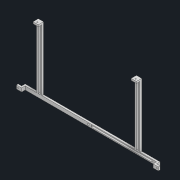
# Autodesk Inventor part: Bancada
Saved by Autodesk Inventor 2021 (Build 250183000, 183)
## iProperties
Created: 2021-04-19
Part Number: Bancada
Material: Genérico
Document SubType Name: Modeling
Designer: carlo
Density: 1 g/cm^3
Appearance: Valor por defecto
Mass: 32.5704 g
Surface Area: 255.981 cm^2
Volume: 32.5704 cm^3
Author: carlo
Autodesk Inventor part; units mm, degrees
ref_plane "YZ Plane" through (0, 0, 0) normal (1, 0, 0) x (0, 1, 0)
ref_plane "XZ Plane" through (0, 0, 0) normal (0, 1, 0) x (-1, 0, 0)
ref_plane "XY Plane" through (0, 0, 0) normal (0, 0, 1) x (1, 0, 0)
sketch "Boceto1" plane through (0, 0, 0) normal (0, 0, 1) x (1, 0, 0)
  line L0 (5, -5) -> (165, -5)
  line L1 (165, -2.5) -> (8, -2.5)
  line L2 (8, -2.5) -> (8, 2.5)
  line L3 (8, 2.5) -> (165, 2.5)
  line L4 (140, 5) -> (142.5, 5)
  line L5 (142.5, 5) -> (137.5, 5)
  line L6 (137.5, 5) -> (137.5, 180)
  line L7 (142.5, 180) -> (142.5, 5)
  line L8 (132.5, 185) -> (147.5, 185)
  line L9 (147.5, 185) -> (147.5, 5)
  line L10 (142.5, 5) -> (137.5, 5)
  line L11 (132.5, 5) -> (132.5, 185)
  line L12 (137.5, 180) -> (142.5, 180)
  line L13 (147.5, 5) -> (165, 5)
  line L14 (0, 5) -> (132.5, 5)
  line L15 (137.5, 5) -> (142.5, 5)
  arc A0 (-165, 5) -> (-165, -5) centre (-165, 0) ccw
  line L16 (5, -5) -> (-165, -5)
  line L17 (-140, 5) -> (-142.5, 5)
  line L18 (-142.5, 5) -> (-137.5, 5)
  line L19 (-137.5, 5) -> (-137.5, 180)
  line L20 (-142.5, 180) -> (-142.5, 5)
  line L21 (-132.5, 185) -> (-147.5, 185)
  line L22 (-147.5, 185) -> (-147.5, 5)
  line L23 (-142.5, 5) -> (-137.5, 5)
  line L24 (-132.5, 5) -> (-132.5, 185)
  line L25 (-137.5, 180) -> (-142.5, 180)
  line L26 (-147.5, 5) -> (-165, 5)
  line L27 (0, 5) -> (-132.5, 5)
  line L28 (-137.5, 5) -> (-142.5, 5)
  line L29 (0, 0) -> (-5, 0) construction
  circle A1 centre (0, 0) radius 2.5
  arc A2 (180, -2.5) -> (180, 2.5) centre (180, 0) ccw
  line L30 (180, 5) -> (165, 5)
  line L31 (165, 2.5) -> (180, 2.5)
  line L32 (165, -2.5) -> (180, -2.5)
  line L33 (165, -5) -> (180, -5)
  arc A3 (180, -5) -> (180, 5) centre (180, 0) ccw
  dimension "d13" = 15
  dimension "d17" = 180
  dimension "d18" = 175
  dimension "d31" = 10
  dimension "d36" = 5
  dimension "d40" = 5
  constraints: 68 end point, 8 parallel, 6 horizontal, 6 point on circle, 4 centre point, 4 perpendicular, 2 coincident, 2 tangent
  measures "d13" distance of L9.end L11.start
  measures "d17" distance of L11.start L8.start
  measures "d18" distance between parallel lines of L14 L12
  measures "d31" distance between parallel lines of L27 L16
  measures "d36" diameter of A1
  measures "d40" diameter of A2
extrude "Extrusión1" add sketch "Boceto1" along normal blind 5
sketch "Sketch4" plane through (0, 0, 5) normal (0, 0, 1) x (1, 0, 0)
  line L0 (-132.5, 185) -> (-147.5, 185) projected
  line L1 (-132.5, 5) -> (-132.5, 185) projected
  line L2 (-147.5, 185) -> (-132.5, 185)
  line L3 (-132.5, 185) -> (-132.5, 180)
  line L4 (-132.5, 180) -> (-147.5, 180)
  line L5 (-147.5, 180) -> (-147.5, 185)
  line L6 (180, 5) -> (147.5, 5) projected
  line L7 (147.5, 5) -> (147.5, 185) projected
  line L8 (147.5, 185) -> (132.5, 185) projected
  line L9 (132.5, 185) -> (132.5, 5) projected
  line L10 (132.5, 5) -> (-132.5, 5) projected
  line L11 (-132.5, 5) -> (-132.5, 185) projected
  line L12 (-132.5, 185) -> (-147.5, 185) projected
  line L13 (-147.5, 185) -> (-147.5, 5) projected
  line L14 (-147.5, 5) -> (-165, 5) projected
  arc A0 (-165, 5) -> (-165, -5) centre (-165, 0) ccw projected
  line L15 (-165, -5) -> (180, -5) projected
  line L16 (-142.5, 5) -> (-142.5, 180) projected
  line L17 (-142.5, 180) -> (-137.5, 180) projected
  line L18 (-137.5, 180) -> (-137.5, 5) projected
  line L19 (-137.5, 5) -> (-142.5, 5) projected
  line L20 (142.5, 180) -> (142.5, 5) projected
  line L21 (142.5, 5) -> (137.5, 5) projected
  line L22 (137.5, 5) -> (137.5, 180) projected
  line L23 (137.5, 180) -> (142.5, 180) projected
  line L24 (132.5, 185) -> (147.5, 185)
  line L25 (147.5, 185) -> (147.5, 180)
  line L26 (147.5, 180) -> (132.5, 180)
  line L27 (132.5, 180) -> (132.5, 185)
  arc A1 (180, -5) -> (180, 5) centre (180, 0) ccw projected
  point P0 (0, 0)
  dimension "d26" = 5
  constraints: 16 end point, 4 parallel, 2 horizontal, 2 perpendicular, 2 point on line
  measures "d26" distance of L2.end L3.end
extrude "Extrusion3" add sketch "Sketch4" along normal blind 10 contours L1 L4 L5 L0 | L9 L8 L7 L26 L23
sketch "Sketch5" plane through (0, 0, 5) normal (0, 0, 1) x (1, 0, 0)
  line L0 (180, -2.5) -> (8, -2.5) projected
  line L1 (8, -2.5) -> (8, 2.5) projected
  line L2 (8, 2.5) -> (180, 2.5) projected
  arc A0 (180, -2.5) -> (180, 2.5) centre (180, 0) ccw projected
  circle A1 centre (0, 0) radius 2.5 projected
  line L3 (147.5, 180) -> (142.5, 180) projected
  line L4 (142.5, 180) -> (142.5, 5) projected
  line L5 (142.5, 5) -> (137.5, 5) projected
  line L6 (137.5, 5) -> (137.5, 180) projected
  line L7 (137.5, 180) -> (132.5, 180) projected
  line L8 (132.5, 180) -> (132.5, 5) projected
  line L9 (132.5, 5) -> (-132.5, 5) projected
  line L10 (-132.5, 5) -> (-132.5, 180) projected
  line L11 (-132.5, 180) -> (-137.5, 180) projected
  line L12 (-137.5, 180) -> (-137.5, 5) projected
  line L13 (-137.5, 5) -> (-142.5, 5) projected
  line L14 (-142.5, 5) -> (-142.5, 180) projected
  line L15 (-142.5, 180) -> (-147.5, 180) projected
  line L16 (-147.5, 180) -> (-147.5, 5) projected
  line L17 (-147.5, 5) -> (-165, 5) projected
  arc A2 (-165, 5) -> (-165, -5) centre (-165, 0) ccw projected
  line L18 (-165, -5) -> (180, -5) projected
  arc A3 (180, -5) -> (180, 5) centre (180, 0) ccw projected
  line L19 (180, 5) -> (147.5, 5) projected
  line L20 (147.5, 5) -> (147.5, 180) projected
  arc A4 (-165, 5) -> (-165, -5) centre (-165, 0) ccw projected
  line L21 (-165, -5) -> (-185, -5)
  line L22 (-185, -5) -> (-185, 5)
  line L23 (-185, 5) -> (-165, 5)
  line L24 (-165, 5) -> (-165, -5)
  arc A5 (180, -5) -> (180, 5) centre (180, 0) ccw projected
  line L25 (180, 5) -> (200, 5)
  line L26 (200, 5) -> (200, -5)
  line L27 (200, -5) -> (180, -5)
  dimension "d42" = 20
  dimension "d45" = 20
  constraints: 14 end point, 3 perpendicular, 2 horizontal, 2 parallel
  measures "d42" distance of L22.end L23.end
  measures "d45" distance of L19.start L25.end
extrude "Extrusion4" add sketch "Sketch5" against normal up to surface (5 mm away) contours L25 L26 L27 A3 | L21 L22 L23 A2 | A2 L24
sketch "Sketch6" plane through (0, 0, 5) normal (0, 0, 1) x (1, 0, 0)
  line L0 (-147.5, 180) -> (-132.5, 180) projected
  line L1 (-132.5, 180) -> (-132.5, 185) projected
  line L2 (-132.5, 185) -> (-147.5, 185) projected
  line L3 (-147.5, 185) -> (-147.5, 180) projected
  line L4 (-147.5, 5) -> (-185, 5) projected
  line L5 (200, -5) -> (-185, -5) projected
  line L6 (-185, 5) -> (-180, 5)
  line L7 (-180, 5) -> (-180, -5)
  line L8 (-180, -5) -> (-185, -5)
  line L9 (-185, -5) -> (-185, 5)
  line L10 (200, -5) -> (200, 5) projected
  line L11 (200, 5) -> (195, 5)
  line L12 (195, 5) -> (195, -5)
  line L13 (195, -5) -> (200, -5)
  line L14 (200, -5) -> (200, 5)
  point P0 (0, 0)
  dimension "d46" = 15
  dimension "d47" = 5
  dimension "d48" = 5
  dimension "d49" = 5
  dimension "d50" = 10
  constraints: 16 end point, 4 parallel, 2 horizontal, 2 perpendicular, 1 point on line
  measures "d46" distance of L1.end L2.end
  measures "d47" distance of L0.end L1.end
  measures "d48" distance of L7.end L8.end
  measures "d49" distance of L13.end L12.end
  measures "d50" distance of L12.end L11.end
extrude "Extrusion5" add sketch "Sketch6" along normal up to surface (10 mm away) contours L7 L5 L9 L4 | L12 L11 L10 L5
sketch "Sketch7" plane through (-185, -5, 0) normal (-1, 0, 0) x (0, 0, 1)
  line L0 (15, 0) -> (15, 10) projected
  line L1 (0, 0) -> (15, 0) projected
  line L2 (15, 10) -> (10, 10)
  line L3 (10, 10) -> (10, 0)
  line L4 (10, 0) -> (15, 0)
  line L5 (15, 0) -> (15, 10)
  point P0 (0, 5)
  dimension "d53" = 5
  constraints: 8 end point, 2 parallel, 1 horizontal, 1 perpendicular, 1 point on line
  measures "d53" distance of L4.end L3.end
extrude "Extrusion6" add sketch "Sketch7" along normal blind 10
sketch "Sketch8" plane through (200, -5, 0) normal (1, 0, 0) x (0, 0, -1)
  line L0 (-10, 10) -> (-10, 0) projected
  line L1 (-10, 0) -> (-15, 0) projected
  line L2 (-15, 0) -> (-15, 10) projected
  line L3 (-15, 10) -> (-10, 10) projected
  point P0 (0, 5)
extrude "Extrusion7" add sketch "Sketch8" along normal blind 10
sketch "Sketch9" plane through (-180, -5, 15) normal (0, 0, 1) x (1, 0, 0)
  line L0 (32.5, 10) -> (-5, 10) projected
  line L1 (0, 0) -> (375, 0) projected
  line L2 (-5, 0) -> (-5, 10) projected
  line L3 (0, 0) -> (-15, 0) projected
  line L4 (0, 10) -> (0, 0) projected
  line L5 (0, 10) -> (-15, 10) projected
  line L6 (-15, 0) -> (-15, 10) projected
  line L7 (-15, 10) -> (-5, 10) construction
  line L8 (-5, 10) -> (-5, 0) construction
  line L9 (-5, 0) -> (-15, 0) construction
  line L10 (-15, 0) -> (-15, 10) construction
  circle A0 centre (-10, 5) radius 1.5
  line L11 (375, 10) -> (390, 10) projected
  line L12 (375, 0) -> (375, 10) projected
  line L13 (375, 0) -> (390, 0) projected
  line L14 (390, 10) -> (390, 0) projected
  line L15 (380, 10) -> (380, 0) projected
  line L16 (327.5, 10) -> (380, 10) construction
  line L17 (375, 0) -> (390, 0) construction
  line L18 (380, 10) -> (390, 10) construction
  line L19 (390, 10) -> (390, 0) construction
  line L20 (390, 0) -> (380, 0) construction
  line L21 (380, 0) -> (380, 10) construction
  circle A1 centre (385, 5) radius 1.5
  point P0 (180, 5)
  dimension "d58" = 3
  dimension "d61" = 3
  constraints: 16 end point, 4 parallel, 2 centre point, 2 horizontal, 2 perpendicular
  measures "d58" diameter of A0
  measures "d61" diameter of A1
extrude "Extrusion8" cut sketch "Sketch9" against normal blind 10 contours A0 | A1
sketch "Sketch10" plane through (-147.5, 185, 0) normal (0, 1, 0) x (1, 0, 0)
  line L0 (342.5, -5) -> (295, -5) projected
  line L1 (295, -5) -> (290, -5) projected
  line L2 (290, -5) -> (285, -5) projected
  line L3 (285, -5) -> (280, -5) projected
  line L4 (280, -5) -> (15, -5) projected
  line L5 (15, -5) -> (10, -5) projected
  line L6 (10, -5) -> (5, -5) projected
  line L7 (5, -5) -> (0, -5) projected
  line L8 (0, -5) -> (-32.5, -5) projected
  line L9 (-32.5, -5) -> (342.5, -5) projected
  line L10 (150, -5) -> (145, -5) projected
  line L11 (327.5, -5) -> (155.5, -5) projected
  line L12 (155.5, -5) -> (327.5, -5) projected
  line L13 (327.5, -5) -> (327.5, -5) projected
  line L14 (15, 0) -> (15, -15) construction
  line L15 (0, -5) -> (15, -5) construction
  line L16 (15, -5) -> (15, -15) construction
  line L17 (15, -15) -> (0, -15) construction
  line L18 (0, -15) -> (0, -5) construction
  line L19 (295, 0) -> (295, -15) construction
  line L20 (295, -15) -> (280, -15) construction
  line L21 (280, -15) -> (280, -5) construction
  line L22 (280, -5) -> (295, -5) construction
  line L23 (295, -5) -> (295, -15) construction
  circle A0 centre (7.5, -10) radius 1.5
  circle A1 centre (287.5, -10) radius 1.5
  point P0 (147.5, 0)
  dimension "d62" = 3
  dimension "d63" = 3
  constraints: 16 end point, 4 parallel, 2 centre point, 2 horizontal, 2 perpendicular
  measures "d62" diameter of A0
  measures "d63" diameter of A1
extrude "Extrusion9" cut sketch "Sketch10" against normal blind 10
